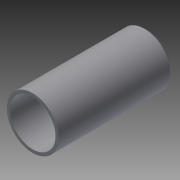
# Autodesk Inventor part: pierscien nr 2 srodkowy v2
Saved by Autodesk Inventor 2014 (Build 180170000, 170)
## iProperties
Created: 2017-04-18
Part Number: pierscien nr 2 srodkowy v2
Material: Ogólny
Document SubType Name: Konstrukcja blachowa
Designer: hpdc7700
Density: 1 g/cm^3
Appearance: Domyślna
Sheet Metal Rule: Domyślny
Author: hpdc7700
Autodesk Inventor part; units mm, degrees
ref_plane "YZ Plane" through (0, 0, 0) normal (1, 0, 0) x (0, 1, 0)
ref_plane "XZ Plane" through (0, 0, 0) normal (0, 1, 0) x (-1, 0, 0)
ref_plane "XY Plane" through (0, 0, 0) normal (0, 0, 1) x (1, 0, 0)
sketch "Szkic1" plane through (0, 0, 0) normal (0, 1, 0) x (-1, 0, 0)
  circle A0 centre (0, 0) radius 7.95
  circle A1 centre (0, 0) radius 9.05
  dimension "d0" = 15.9
  dimension "d1" = 18.1
  constraints: 2 centre point, 2 coincident
  measures "d0" diameter of A0
  measures "d1" diameter of A1
extrude "Wyciągnięcie proste1" add sketch "Szkic1" along normal blind 40
chamfer "Faza1" distance 1 angle 45 1 edges at (9.05, 40, 0)
equation "\"PromieńGięcia\" = Grubość"
equation "\"SzerokośćGięciaPodcięcia\" = Grubość"
equation "\"GłębokośćGięciaPodcięcia\" = 0.5 * Grubość"
equation "\"RozmiarPodcięciaNarożnika\" = 4 * Grubość"
equation "\"MinimalnaPozostałość\" = 2 * Grubość"
equation "\"PromieńPrzejścia\" = PromieńGięcia"
equation "\"Rozmiar_promienia_Jacobiego\" = Grubość"
equation "\"Wielk_odstępu\" = Grubość"
equation "\"Grubość\" = 0.5"
